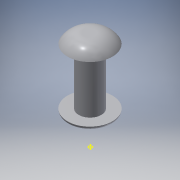
# Autodesk Inventor part: MS20470 A 2-4
Saved by Autodesk Inventor 2018 (Build 220105000, 105)
## iProperties
Created: 2004-10-19
Part Number: MS20470 A 2-4
Document SubType Name: Modeling
Designer: Autodesk, Inc.
Manufacturer: Standard
Standards Organization: Custom
Material: Aluminum-6061
Description: #2 x 0.25 RIVET, SOLID, UNIVERSAL HEAD
Mass: 0.0360393 g
Surface Area: 0.509577 cm^2
Volume: 0.0132986 cm^3
Density: 2.71 g/cm^3
Appearance: Aluminum - Flat
CAGE: 1LJX3
Dept. ID: Product Design
Description #2: ---
Finish #1: ---
Finish #2: ---
Material ID: ---
Project Number: ---
Author: Autodesk, Inc.
Autodesk Inventor part; units mm, degrees
ref_plane "YZ Plane" through (0, 0, 0) normal (1, 0, 0) x (0, 1, 0)
ref_plane "XZ Plane" through (0, 0, 0) normal (0, 1, 0) x (-1, 0, 0)
ref_plane "XY Plane" through (0, 0, 0) normal (0, 0, 1) x (1, 0, 0)
sketch "Sketch1" plane through (0, 0, 0) normal (0, 0, 1) x (1, 0, 0)
  circle A0 centre (0, 0) radius 0.8001
  dimension "d0" = 1.6002
  constraints: 1 centre point
  measures "d0" diameter of A0
extrude "Body" add sketch "Sketch1" against normal blind 3.9624
sketch "Sketch2" plane through (0, 0, 0) normal (1, 0, 0) x (0, 1, 0)
  line L0 (-0.328, 0) -> (1.9681, 0) construction
  line L1 (0, -6.8275) -> (0, -3.4849) construction
  line L2 (0, -3.9624) -> (1.5875, -3.9624)
  line L3 (1.5875, -3.9624) -> (1.5875, -3.9624)
  line L4 (1.3335, -4.2164) -> (0, -4.2164)
  line L5 (0, -4.2164) -> (0, -3.9624)
  arc A0 (1.3335, -4.2164) -> (1.5875, -3.9624) centre (1.3335, -3.9624) ccw
  point P0 (1.5875, -4.2164)
  point P1 (0, -6.35)
  dimension "d3" = 3.9624
  dimension "d4" = 3.175
  dimension "d5" = 0.254
  dimension "d6" = 0.254
  dimension "d11" = 6.35
  constraints: 8 end point, 4 point on line, 2 parallel, 2 point on circle, 2 tangent, 1 centre point, 1 horizontal, 1 perpendicular
  measures "d3" distance between parallel lines of L2 L0
  measures "d4" diameter of L3 L1
  measures "d5" distance of L2.end point (1.587, -4.216)
  measures "d6" radius of A0
  measures "d11" distance from line of point (0, -6.35) L0
revolve "Deformation" add sketch "Sketch2" angle 360 about axis through (0, 0, -10) along (0, 0, 1)
sketch "Sketch4" plane through (0, 0, 0) normal (1, 0, 0) x (0, 1, 0)
  line L0 (-0.3175, 0) -> (1.905, 0) construction
  line L1 (0, -4.7549) -> (0, 0.7925) projected
  line L2 (0, 0) -> (1.5875, 0)
  line L3 (1.5875, 0) -> (1.5875, -0.1016)
  line L4 (1.5875, -0.1016) -> (0.8001, -0.7623)
  line L5 (0.8001, -0.7623) -> (0, -0.7623)
  line L6 (0.8001, 0) -> (0.8001, -3.9624) construction
  dimension "d12" = 3.175
  dimension "d13" = 0.1016
  dimension "d14" = 50
  dimension "d22" = 0.6607
  constraints: 8 end point, 5 point on line, 2 perpendicular
  measures "d12" diameter of L3 L1
  measures "d13" distance of L2.end L3.end
  measures "d14" angle of L1 L4
  measures "d22" distance from line of L5 L3.end
revolve "CSink Head" [suppressed]
sketch "Sketch5" plane through (0, 0, 0) normal (1, 0, 0) x (0, 1, 0)
  line L0 (0, -0.9919) -> (0, 1.1511) projected
  line L1 (-0.3347, 0) -> (2.0081, 0) construction
  line L2 (0, 0.6858) -> (0.3937, 0.6858)
  arc A0 (1.5815, 0) -> (0.3937, 0.6858) centre (0.3937, -0.6858) ccw
  line L3 (1.5815, 0) -> (0, 0)
  dimension "d16" = 0.7874
  dimension "d17" = 1.3716
  dimension "d18" = 0.3937
  dimension "d19" = 0.6858
  constraints: 4 end point, 4 point on line, 2 point on circle, 1 centre point, 1 parallel, 1 tangent
  measures "d16" diameter of L2.end L0
  measures "d17" radius of A0
  measures "d18" distance from line of A0.centre L0
  measures "d19" distance between parallel lines of L2 L1
revolve "Universal Head" add sketch "Sketch5" angle 360 about axis through (0, 0, -10) along (0, 0, 1)
equation "\"d0\" = Dim_D"
equation "\"d1\" = Engage_Length"
equation "\"d3\" = Engage_Length"
equation "\"d4\" = Dim_A"
equation "\"d5\" = 0.5 * Dim_T"
equation "\"d6\" = d5"
equation "\"d11\" = Length"
equation "\"d12\" = Dim_A"
equation "\"d13\" = Dim_E_CSink"
equation "\"d16\" = Dim_E_Univ"
equation "\"d17\" = Dim_R"
equation "\"d19\" = Dim_C"
equation "\"Dim_A\" = 3.175"
equation "\"Dim_B\" = 2.3876"
equation "\"Dim_C_CSink\" = Dim_B"
equation "\"Dim_D\" = 1.6002"
equation "\"Dim_E_CSink\" = 0.1016"
equation "\"Dim_S\" = 0.5842"
equation "\"Dim_T\" = 0.508"
equation "\"Engage_Length\" = Length - Dim_C_CSink"
equation "\"Length\" = 6.35"
equation "\"Dim_E_Univ\" = 0.7874"
equation "\"Dim_F\" = 0.5842"
equation "\"Dim_R\" = 1.3716"
equation "\"Dim_C\" = 0.6858"
body "Solid1"
